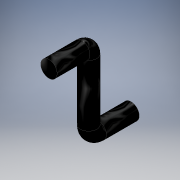
# Autodesk Inventor part: crank bar
Saved by Autodesk Inventor 2018 (Build 220112000, 112)
## iProperties
Created: 2018-10-03
Part Number: crank bar
Material: ABS Plastic
Document SubType Name: Modeling
Designer: Jayden
Density: 1.06 g/cm^3
Appearance: Black
Author: Jayden
Autodesk Inventor part; units mm, degrees
ref_plane "YZ Plane" through (0, 0, 0) normal (1, 0, 0) x (0, 1, 0)
ref_plane "XZ Plane" through (0, 0, 0) normal (0, 1, 0) x (-1, 0, 0)
ref_plane "XY Plane" through (0, 0, 0) normal (0, 0, 1) x (1, 0, 0)
sketch "Sketch3" plane through (0, 0, 0) normal (0, 0, 1) x (1, 0, 0)
  circle A0 centre (0, 7.5) radius 1.5875
  point P0 (0, 0)
  dimension "d10" = 3.175
  dimension "d11" = 7.5
  constraints: 1 centre point
  measures "d10" diameter of A0
  measures "d11" distance of A0.centre point (0, 0)
sketch "Sketch4" plane through (0, 0, 0) normal (1, 0, 0) x (0, 1, 0)
  line L0 (7.7682, 0) -> (7.7682, -6.35)
  line L1 (7.7682, 0) -> (14.1182, 0) construction
  line L2 (6.1807, -7.9375) -> (-5.6443, -7.9375)
  line L3 (-7.2318, -9.525) -> (-7.2318, -15.875)
  arc A0 (6.1807, -7.9375) -> (7.7682, -6.35) centre (6.1807, -6.35) ccw
  arc A1 (-5.6443, -7.9375) -> (-7.2318, -9.525) centre (-5.6443, -9.525) ccw
  point P0 (0, 0)
  point P1 (7.7682, -7.9375)
  point P2 (-7.2318, -7.9375)
  dimension "d12" = 7.9375
  dimension "d13" = 90
  dimension "d14" = 15
  dimension "d15" = 90
  dimension "d16" = 7.9375
  dimension "d17" = 1.5875
  constraints: 8 end point, 4 point on circle, 4 point on line, 4 tangent, 3 perpendicular, 2 centre point, 1 equal radius, 1 horizontal, 1 vertical
  measures "d12" distance of L0.start point (7.768, -7.938)
  measures "d13" angle of L0 L1
  measures "d14" distance of point (7.768, -7.938) point (-7.232, -7.938)
  measures "d15" angle of L0 L2
  measures "d16" distance of point (-7.232, -7.938) L3.end
  measures "d17" radius of A0
sweep "Sweep2" add profiles "Sketch3" path "Sketch4"
body "Solid2"
